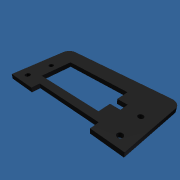
# Autodesk Inventor part: Acrylic_YawServoSupport_2
Saved by Autodesk Inventor 2012 (Build 160160000, 160)
## iProperties
Created: 2014-03-29
Part Number: Acrylic_YawServoSupport_2
Material: Default
Document SubType Name: Modeling
Designer: Admin
Density: 1 g/cm^3
Author: Admin
Autodesk Inventor part; units mm, degrees
ref_plane "YZ Plane" through (0, 0, 0) normal (1, 0, 0) x (0, 1, 0)
ref_plane "XZ Plane" through (0, 0, 0) normal (0, 1, 0) x (-1, 0, 0)
ref_plane "XY Plane" through (0, 0, 0) normal (0, 0, 1) x (1, 0, 0)
sketch "Sketch1" plane through (0, 0, 0) normal (0, 0, 1) x (1, 0, 0)
  line L0 (-53.9497, 0) -> (53.9497, 0) projected
  line L1 (0, -8.2071) -> (0, 49.2426) projected
  line L2 (-37.5, 0) -> (37.5, 0)
  line L3 (37.5, 0) -> (37.5, 35)
  line L4 (32.5, 40) -> (-32.5, 40)
  line L5 (-37.5, 35) -> (-37.5, 0)
  arc A0 (-32.5, 40) -> (-37.5, 35) centre (-32.5, 35) ccw
  arc A1 (37.5, 35) -> (32.5, 40) centre (32.5, 35) ccw
  point P0 (0, 0)
  point P1 (37.5, 40)
  point P2 (-37.5, 40)
  dimension "d0" = 75
  dimension "d1" = 40
  dimension "d2" = 37.5
  dimension "d5" = 5
  constraints: 8 end point, 5 point on line, 4 point on circle, 4 tangent, 2 centre point, 2 parallel, 1 equal radius, 1 horizontal, 1 perpendicular
  measures "d0" distance of point (-37.5, 40) point (37.5, 40)
  measures "d1" distance of point (37.5, 40) L2.end
  measures "d2" distance between parallel lines of L5 L1
  measures "d5" radius of A0
extrude "Extrusion1" add sketch "Sketch1" along normal blind 2.8
sketch "Sketch2" plane through (0, 0, 0) normal (0, 0, -1) x (-1, 0, 0)
  line L0 (37.5, 0) -> (-37.5, 0) projected
  line L1 (-20, 0) -> (-20, 5)
  line L2 (-20, 5) -> (20, 5)
  line L3 (20, 5) -> (20, 0)
  line L4 (-15.15, 22.4) -> (-21.15, 22.4)
  line L5 (-21.15, 22.4) -> (-21.15, 17.4)
  line L6 (-21.15, 17.4) -> (-15.15, 17.4)
  line L7 (-15.15, 17.4) -> (-15.15, 10)
  line L8 (25.15, 29.8) -> (-15.15, 29.8)
  line L9 (-15.15, 10) -> (25.15, 10)
  line L10 (25.15, 10) -> (25.15, 29.8)
  line L11 (-37.5, 0) -> (-37.5, 35) projected
  line L12 (-15.15, 22.4) -> (-15.15, 29.8)
  circle A0 centre (-30, 20) radius 1.5
  circle A1 centre (30, 20) radius 1.5
  arc A2 (-29.5144, 4.6) -> (-29.3, 5.4) centre (-30.9, 5.4) ccw
  line L13 (-32.5, 40) -> (32.5, 40) projected
  line L14 (-32.5, 5.4) -> (-32.5, 7)
  line L15 (-29.3, 7) -> (-29.3, 3.8)
  line L16 (-32.5, 3.8) -> (-32.5, 5.4)
  arc A3 (-29.3, 7) -> (-32.5, 7) centre (-30.9, 7) ccw
  arc A4 (-32.5, 3.8) -> (-29.3, 3.8) centre (-30.9, 3.8) ccw
  line L17 (37.5, 35) -> (37.5, 0) projected
  line L18 (29.3, 5.4) -> (29.3, 7)
  line L19 (32.5, 7) -> (32.5, 3.8)
  line L20 (29.3, 3.8) -> (29.3, 5.4)
  arc A5 (32.5, 7) -> (29.3, 7) centre (30.9, 7) ccw
  arc A6 (29.3, 3.8) -> (32.5, 3.8) centre (30.9, 3.8) ccw
  point P0 (0, 0)
  dimension "d9" = 3.2
  dimension "d10" = 3.2
  dimension "d13" = 3.2
  dimension "d14" = 3.2
  constraints: 34 end point, 10 point on circle, 7 centre point, 5 horizontal, 5 parallel, 5 vertical, 1 collinear, 1 midpoint, 1 perpendicular, 1 tangent, 18 other
  measures "d9" diameter of A3
  measures "d10" diameter of A4
  measures "d13" diameter of A5
  measures "d14" diameter of A6
extrude "Extrusion2" cut sketch "Sketch2" against normal blind 10
equation "\"d2\" = 0.5 * d0"
body "Solid1"
